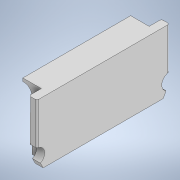
# Autodesk Inventor part: USB-Deckel
Saved by Autodesk Inventor 2021.1 (Build 251245010, 245A)
## iProperties
Created: 2021-02-18
Part Number: USB-Deckel
Material: Generisch
Document SubType Name: Modeling
Designer: hpcthobs
Density: 1 g/cm^3
Appearance: Vorgabe
Author: hpcthobs
Autodesk Inventor part; units mm, degrees
ref_plane "YZ Plane" through (0, 0, 0) normal (1, 0, 0) x (0, 1, 0)
ref_plane "XZ Plane" through (0, 0, 0) normal (0, 1, 0) x (-1, 0, 0)
ref_plane "XY Plane" through (0, 0, 0) normal (0, 0, 1) x (1, 0, 0)
sketch "Skizze1" plane through (0, 0, 0) normal (0, 1, 0) x (-1, 0, 0)
  line L0 (0, 0) -> (1.3, 0)
  line L1 (1.3, 0) -> (1.3, -21.5)
  line L2 (1.3, -21.5) -> (0, -21.5)
  line L3 (0, -21.5) -> (0, 0)
  line L4 (1.3, 0) -> (2.8, 0)
  line L5 (2.8, 0) -> (2.8, -21.5)
  line L6 (2.8, -21.5) -> (1.3, -21.5)
  line L7 (1.3, -21.5) -> (1.3, 0)
  line L8 (2.8, 0) -> (1.3, 0)
  line L9 (1.3, 0) -> (1.3, -2)
  line L10 (1.3, -2) -> (2.8, -2)
  line L11 (2.8, -2) -> (2.8, 0)
  line L12 (1.3, -21.5) -> (2.8, -21.5)
  line L13 (2.8, -21.5) -> (2.8, -19.5)
  line L14 (2.8, -19.5) -> (1.3, -19.5)
  line L15 (1.3, -19.5) -> (1.3, -21.5)
  point P0 (1.3, -19.5)
  point P1 (2.8, -2)
  point P2 (1.3, -2)
  dimension "d0" = 1.3
  dimension "d1" = 21.5
  dimension "d2" = 1.5
  dimension "d3" = 2
  dimension "d4" = 2
  constraints: 32 end point, 8 parallel, 4 horizontal, 4 perpendicular, 2 point on line
  measures "d0" distance of L1.end L2.end
  measures "d1" distance of L0.end L1.end
  measures "d2" distance of L5.end L6.end
  measures "d3" distance of L9.end L8.end
  measures "d4" distance of L13.end L12.end
extrude "Extrusion1" add sketch "Skizze1" along normal blind 10 contours L0 L1 L2 L3 | L10 L5 L14 L1
sketch "Skizze3" plane through (-2.8, 0, -19.5) normal (-1, 0, 0) x (0, 0, 1)
  line L0 (12.2393, 3.0088) -> (12.2393, 2.4088)
  line L1 (12.2393, 2.4088) -> (10.2953, 2.4088)
  arc A0 (9.9169, 2.6153) -> (10.2953, 2.4088) centre (10.2953, 2.8588) ccw
  line L2 (9.9169, 2.6153) -> (8.6983, 4.5088)
  line L3 (8.6983, 4.5088) -> (15.3893, 4.5088)
  line L4 (15.3893, 4.5088) -> (15.3893, 3.9088)
  line L5 (15.3893, 3.9088) -> (16.9481, 4.8088)
  line L6 (16.9481, 4.8088) -> (15.3893, 5.7088)
  line L7 (15.3893, 5.7088) -> (15.3893, 5.1088)
  line L8 (15.3893, 5.1088) -> (6.148, 5.1088)
  line L9 (6.148, 5.1088) -> (7.3604, 7.0016)
  arc A1 (7.7393, 7.2088) -> (7.3604, 7.0016) centre (7.7393, 6.7588) ccw
  line L10 (7.7393, 7.2088) -> (10.0408, 7.2088)
  arc A2 (10.0408, 7.2088) -> (10.0408, 7.8088) centre (10.8893, 7.5088) ccw
  line L11 (10.0408, 7.8088) -> (7.7393, 7.8088)
  arc A3 (7.7393, 7.8088) -> (6.8551, 7.3252) centre (7.7393, 6.7588) ccw
  line L12 (6.8551, 7.3252) -> (5.5682, 5.3161)
  arc A4 (5.1893, 5.1088) -> (5.5682, 5.3161) centre (5.1893, 5.5588) ccw
  line L13 (5.1893, 5.1088) -> (3.959, 5.1088)
  arc A5 (3.959, 5.1088) -> (3.959, 4.5088) centre (2.4893, 4.8088) ccw
  line L14 (3.959, 4.5088) -> (7.7393, 4.5088)
  arc A6 (8.1177, 4.3024) -> (7.7393, 4.5088) centre (7.7393, 4.0588) ccw
  line L15 (8.1177, 4.3024) -> (9.4123, 2.2906)
  arc A7 (9.4123, 2.2906) -> (10.2953, 1.8088) centre (10.2953, 2.8588) ccw
  line L16 (10.2953, 1.8088) -> (12.2393, 1.8088)
  line L17 (12.2393, 1.8088) -> (12.2393, 1.2088)
  line L18 (12.2393, 1.2088) -> (14.0393, 1.2088)
  line L19 (14.0393, 1.2088) -> (14.0393, 3.0088)
  line L20 (14.0393, 3.0088) -> (12.2393, 3.0088)
  point P0 (19.5, 0)
  point P1 (8.1177, 4.3024)
  point P2 (9.4123, 2.2906)
  point P3 (10.2953, 1.8088)
  point P4 (9.9169, 2.6153)
  point P5 (6.148, 5.1088)
  point P6 (7.3604, 7.0016)
  point P7 (7.7393, 7.2088)
  point P8 (10.0408, 7.8088)
  point P9 (7.7393, 7.8088)
  point P10 (6.8551, 7.3252)
  point P11 (5.1893, 5.1088)
  point P12 (3.959, 5.1088)
  point P13 (3.959, 4.5088)
  point P14 (7.7393, 4.5088)
  constraints: 42 end point, 16 point on circle, 8 centre point
extrude "Extrusion2" add sketch "Skizze3" along normal blind 0.4
sketch "Skizze4" plane through (-2.8, 0, -2) normal (0, 0, 1) x (1, 0, 0)
  line L0 (1.5, 10) -> (0, 10) projected
  line L1 (0, 10) -> (-1.5, 10)
  line L2 (0, 10) -> (-1.5, 10)
  line L3 (-1.5, 10) -> (-1.5, 9.5)
  line L4 (-1.5, 9.5) -> (0, 9.5)
  line L5 (0, 9.5) -> (0, 10)
  line L6 (0, 9.5) -> (0, 8)
  line L7 (0, 7.8088) -> (-0.4, 7.8088) projected
  line L8 (-1.5, 9.5) -> (0, 9.5) construction
  line L9 (0, 9.5) -> (0, 7.8088) construction
  line L10 (0, 0) -> (0, 10) projected
  spline S0 degree 2 poles (-1.5, 9.5) (0, 9.5) (0, 7.8088) knots 1 1 1 2 2 2
  point P0 (2.8, 0)
  dimension "d9" = 1.5
  dimension "d10" = 0.5
  dimension "d11" = 1.5
  constraints: 12 end point, 3 perpendicular, 2 horizontal, 2 parallel, 1 coincident, 1 collinear, 3 other
  measures "d9" distance of L0.end L1.end
  measures "d10" distance of L3.end L2.end
  measures "d11" distance of L4.end L6.end
extrude "Extrusion3" add sketch "Skizze4" against normal up to surface (17.5 mm away)
sketch "Skizze5" plane through (-1.3, 0, -2) normal (-1, 0, 0) x (0, 0, 1)
  line L0 (0, 10) -> (2, 10) projected
  line L1 (2, 10) -> (2, 2)
  line L2 (2, 0) -> (2, 10) projected
  line L3 (2, 2) -> (-19.5, 2)
  line L4 (-19.5, 0) -> (-19.5, 10) projected
  circle A0 centre (2, 2) radius 1.25
  circle A1 centre (-19.5, 2) radius 1.25
  line L5 (2, 0) -> (-19.5, 0) projected
  line L6 (1, 0) -> (2, 2)
  line L7 (-19.5, 0) -> (-17.5, 0) projected
  line L8 (-18.5, 0) -> (-19.5, 2)
  point P0 (1.441, 0.882)
  point P1 (2, 0.75)
  point P2 (-18.5, 0)
  point P3 (-18.941, 0.882)
  point P4 (-19.5, 0.75)
  dimension "d14" = 8
  dimension "d15" = 2.5
  dimension "d16" = 2.5
  constraints: 8 end point, 3 point on line, 2 centre point, 2 coincident, 1 midpoint, 1 perpendicular
  measures "d14" distance of L0.end L1.end
  measures "d15" diameter of A0
  measures "d16" diameter of A1
extrude "Extrusion4" cut sketch "Skizze5" against normal up to surface (1.3 mm away) contours A0 L2 L1 | L1 L3 A0 | L6 A0 L3 | L2 A0 L6 | L2 L5 L6 A0 | A1 L8 L3 | L3 L4 A1 | L8 A1 L4 | L4 A1 | L8 L5 L4 A1
fillet "Rundung1" radius 0.3 4 edges at (-1.3, 6.625, 0) (-1.3, 6.625, -21.5) (0, 6.625, -21.5) (0, 6.625, 0)
